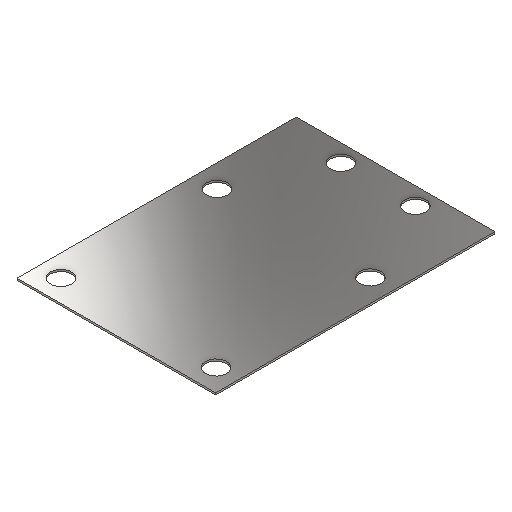
# Autodesk Inventor part: B_holder_sub_muti-holes
Saved by Autodesk Inventor 2026.2 (Build 302298000, 298)
## iProperties
Created: 2026-02-20
Part Number: B_holder_sub_muti-holes
Material: ステンレス鋼 440C
Document SubType Name: Modeling
Designer: zetsu
Density: 7.75 g/cm^3
Appearance: 半つや出し
Author: zetsu
Autodesk Inventor part; units mm, degrees
ref_plane "YZ Plane" through (0, 0, 0) normal (1, 0, 0) x (0, 1, 0)
ref_plane "XZ Plane" through (0, 0, 0) normal (0, 1, 0) x (-1, 0, 0)
ref_plane "XY Plane" through (0, 0, 0) normal (0, 0, 1) x (1, 0, 0)
sketch "スケッチ1" plane through (0, 0, 0) normal (0, 1, 0) x (-1, 0, 0)
  line L0 (16, -31) -> (16, 14)
  line L1 (16, 14) -> (-16, 14)
  line L2 (-16, 14) -> (-16, -31)
  line L3 (-16, -31) -> (16, -31)
  line L4 (0, 0) -> (0, -32.6995) construction
  point P0 (0, 14)
  dimension "d0" = 45
  dimension "d1" = 32
  dimension "d2" = 14
  constraints: 10 end point, 3 perpendicular, 2 vertical, 1 midpoint, 1 other
  measures "d0" distance of L0.end L0.start
  measures "d1" distance of L1.end L0.end
  measures "d2" distance of point (0, 14) L4.start
extrude "押し出し1" add sketch "スケッチ1" along normal blind 0.3
sketch "スケッチ4" plane through (0, 0.3, 0) normal (0, 1, 0) x (1, 0, 0)
  line L0 (0, 0) -> (-18.7084, 0) construction
  circle A0 centre (-6, 28.2) radius 1.7
  circle A1 centre (6, 28.2) radius 1.7
  line L1 (0, 0) -> (0, 29.6633) construction
  line L2 (16, 31) -> (-16, 31) projected
  point P0 (0, 31)
  dimension "d35" = 3.4
  dimension "d36" = 3.4
  dimension "d37" = 6
  dimension "d38" = 2.8
  constraints: 4 end point, 2 centre point, 1 horizontal, 1 midpoint, 1 symmetric about line, 1 vertical
  measures "d35" diameter of A0
  measures "d36" diameter of A1
  measures "d37" horizontal distance of A1.centre L0.start
  measures "d38" vertical distance of point (0, 31) A1.centre
extrude "押し出し3" cut sketch "スケッチ4" against normal through all
sketch "スケッチ7" plane through (0, 0.3, 0) normal (0, 1, 0) x (1, 0, 0)
  circle A0 centre (-12.5, -10.4296) radius 1.7
  circle A1 centre (12.5, -10.4296) radius 1.7
  circle A2 centre (12.3554, 14.5704) radius 1.7
  circle A3 centre (-12.3554, 14.5704) radius 1.7
  line L0 (0, 0) -> (0, 34.4459) construction
  dimension "d47" = 3.4
  dimension "d48" = 3.4
  dimension "d49" = 3.4
  dimension "d50" = 3.4
  dimension "d51" = 25
  dimension "d52" = 25
  constraints: 4 centre point, 2 end point, 2 symmetric about line, 1 vertical
  measures "d47" diameter of A0
  measures "d48" diameter of A1
  measures "d49" diameter of A2
  measures "d50" diameter of A3
  measures "d51" distance of A1.centre A0.centre
  measures "d52" vertical distance of A1.centre A2.centre
extrude "押し出し6" cut sketch "スケッチ7" against normal through all
